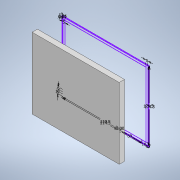
# Autodesk Inventor part: controller_box
Saved by Autodesk Inventor 2022 (Build 260153000, 153)
## iProperties
Created: 2021-07-22
Part Number: controller_box
Material: Generic
Document SubType Name: Modeling
Designer: alibe
Density: 1 g/cm^3
Appearance: Default
Author: alibe
Autodesk Inventor part; units mm, degrees
ref_plane "YZ Plane" through (0, 0, 0) normal (1, 0, 0) x (0, 1, 0)
ref_plane "XZ Plane" through (0, 0, 0) normal (0, 1, 0) x (-1, 0, 0)
ref_plane "XY Plane" through (0, 0, 0) normal (0, 0, 1) x (1, 0, 0)
sketch "Base" plane through (0, 0, 0) normal (0, 0, 1) x (1, 0, 0)
  line L0 (-100, 100) -> (-100, -50)
  line L1 (100, 100) -> (100, -50)
  line L2 (-100, 100) -> (-100, 110)
  line L3 (-100, 110) -> (100, 110)
  line L4 (100, 110) -> (100, 100)
  line L5 (-100, 110) -> (-105, 110)
  line L6 (-105, 110) -> (-105, -50)
  line L7 (-105, -50) -> (-100, -50)
  line L8 (-105, -50) -> (-105, -45)
  line L9 (100, 110) -> (100, 105)
  line L10 (100, 105) -> (-105, 105)
  line L11 (100, 110) -> (105, 110)
  line L12 (105, 110) -> (105, -50)
  line L13 (-105, -50) -> (-105, -60)
  line L14 (-105, -60) -> (105, -60)
  line L15 (105, -60) -> (105, -50)
  line L16 (-105, -60) -> (-105, -55)
  line L17 (-105, -55) -> (105, -55)
  line L18 (100, -50) -> (100, -55)
  line L19 (-100, -50) -> (-100, -55)
  line L20 (-100, -55) -> (-90, -55)
  line L21 (-90, -55) -> (-90, -60)
  line L22 (100, -55) -> (90, -55)
  line L23 (90, -55) -> (90, -60)
  line L24 (-90, -55) -> (-30, -55)
  line L25 (-30, -55) -> (-30, -60)
  line L26 (90, -55) -> (30, -55)
  line L27 (30, -55) -> (30, -60)
  line L28 (-30, -55) -> (-30, 0)
  line L29 (-90, -55) -> (-90, 0)
  line L30 (-90, 0) -> (-30, 0)
  line L31 (30, -55) -> (30, 0)
  line L32 (30, 0) -> (90, 0)
  line L33 (90, 0) -> (90, -55)
  line L34 (-30, -55) -> (-28, -55)
  line L35 (-28, -55) -> (-28, 0)
  line L36 (30, -55) -> (28, -55)
  line L37 (28, -55) -> (28, 0)
  line L38 (-60, -55) -> (-60, 0)
  line L39 (0, 105) -> (0, -55)
  line L40 (-60, 0) -> (-80, 0)
  line L41 (-80, 0) -> (-80, -55)
  line L42 (-60, -55) -> (-40, -55)
  line L43 (-40, -55) -> (-40, 0)
  line L44 (60, -55) -> (60, 0)
  line L45 (80, 0) -> (80, -55)
  line L46 (40, -55) -> (40, 0)
  line L47 (90, -55) -> (95, -55)
  line L48 (80, 0) -> (85, 0)
  line L49 (85, 0) -> (85, -55)
  line L50 (40, -55) -> (35, -55)
  line L51 (35, -55) -> (35, 0)
  line L52 (-85, 0) -> (-85, -55)
  line L53 (-35, -55) -> (-35, 0)
  line L54 (-90, -55) -> (-90, -50)
  line L55 (90, -55) -> (90, -45)
  line L56 (90, -45) -> (28, -45)
  line L57 (-28, -55) -> (-28, -45)
  line L58 (-28, -45) -> (-90, -45)
  line L59 (-90, -45) -> (-90, -35)
  line L60 (-90, -35) -> (-28, -35)
  line L61 (28, -45) -> (28, -35)
  line L62 (28, -35) -> (90, -35)
  point P0 (0, 0)
  point P1 (-100, 105)
  point P2 (-35, -45)
  point P3 (-85, -45)
  point P4 (85, -45)
  point P5 (35, -45)
  point P6 (-85, -35)
  point P7 (-35, -35)
  point P8 (35, -35)
  point P9 (85, -35)
  dimension "d7" = 10
  dimension "d8" = 5
  dimension "d9" = 5
  dimension "d11" = 5
  dimension "d12" = 10
  dimension "d13" = 5
  dimension "d14" = 10
  dimension "d15" = 10
  dimension "d16" = 60
  dimension "d17" = 60
  dimension "d18" = 90
  dimension "d19" = 2
  dimension "d20" = 2
  dimension "d21" = 20
  dimension "d22" = 20
  dimension "d25" = 5
  dimension "d26" = 5
  dimension "d145" = 10
  dimension "d146" = 10
  constraints: 124 end point, 28 point on line, 20 perpendicular, 10 symmetric about line, 8 vertical, 6 midpoint, 1 horizontal, 1 parallel, 12 other
  measures "d7" distance of L0.start L2.end
  measures "d8" distance of L2.end L5.end
  measures "d9" distance of L6.end L8.end
  measures "d11" distance of L3.end L11.end
  measures "d12" distance of L6.end L13.end
  measures "d13" distance of L13.end L16.end
  measures "d14" distance of L19.end L20.end
  measures "d15" distance of L18.end L22.end
  measures "d16" distance of L20.end L24.end
  measures "d17" distance of L22.end L26.end
  measures "d18" angle of L27 L26
  measures "d19" distance of L24.end L34.end
  measures "d20" distance of L26.end L36.end
  measures "d21" distance of L38.end L40.end
  measures "d22" distance of L38.start L42.end
  measures "d25" distance of L45.start L48.end
  measures "d26" distance of L46.start L50.end
  measures "d145" distance of L58.end L59.end
  measures "d146" distance of L56.end L61.end
extrude "base_extrusion" add sketch "Base" against normal blind 3
extrude "wall_extrusion" add sketch "Base" along normal blind 70 contours L0 L7 L6 L10 L2 | L19 L17 L13 L7 | L10 L6 L5 L2 | L2 L3 L4 L10 | L17 L21 L14 L13 | L17 L25 L14 L21 | L11 L12 L15 L17 L18 L1 L4 | L17 L27 L14 L25 | L17 L23 L14 L27 | L15 L14 L23 L17
sketch "pump_holder" plane through (-105, -60, -3) normal (0, -1, 0) x (1, 0, 0)
  line L0 (210, 0) -> (0, 0) projected
  line L1 (0, 73) -> (210, 73)
  line L2 (210, 73) -> (210, 0)
  line L3 (210, 0) -> (0, 0)
  line L4 (0, 0) -> (0, 73)
  line L5 (0, 0) -> (0, 73) projected
  line L6 (0, 0) -> (0, 3)
  line L7 (0, 3) -> (210, 3)
  line L8 (210, 73) -> (210, 0) projected
  line L9 (0, 3) -> (5, 3)
  line L10 (5, 3) -> (5, 0)
  line L11 (5, 3) -> (15, 3)
  line L12 (5, 3) -> (15, 3) construction
  line L13 (15, 3) -> (15, 0)
  line L14 (15, 3) -> (75, 3)
  line L15 (15, 3) -> (75, 3) construction
  line L16 (75, 3) -> (75, 0)
  line L17 (75, 0) -> (77, 0)
  line L18 (15, 0) -> (45, 0)
  line L19 (45, 0) -> (45, 8)
  arc A0 (25, 28) -> (65, 28) centre (45, 28) ccw projected
  line L20 (45, 8) -> (45, 28)
  circle A1 centre (45, 28) radius 20
  line L21 (105, 3) -> (105, 0)
  line L22 (45, 8) -> (45, 10.25)
  line L23 (45, 8) -> (47.25, 8) construction
  line L24 (45, 10.25) -> (74, 10.25)
  line L25 (45, 10.25) -> (73.875, 10.25)
  line L26 (73.875, 10.25) -> (73.875, 55)
  line L27 (73.875, 10.25) -> (118.625, 10.25) construction
  line L28 (73.875, 55) -> (16.125, 55)
  line L29 (73.875, 55) -> (131.625, 55) construction
  line L30 (16.125, 55) -> (16.125, 10.25)
  line L31 (16.125, 10.25) -> (45, 10.25)
  line L32 (45, 28) -> (65, 28)
  line L33 (16.125, 55) -> (16.125, 52)
  line L34 (16.125, 52) -> (19.125, 52)
  line L35 (19.125, 52) -> (20.875, 52)
  line L36 (19.125, 52) -> (20.875, 52) construction
  line L37 (20.875, 52) -> (20.875, 50.25)
  line L38 (20.875, 52) -> (22.625, 52) construction
  line L39 (16.125, 10.25) -> (16.125, 32.625)
  line L40 (16.125, 32.625) -> (21.625, 32.625)
  line L41 (105, 3) -> (105, 73)
  line L42 (205, 73) -> (5, 73) projected
  line L43 (105, 3) -> (175, 3) construction
  line L44 (16.125, 10.25) -> (16.125, 3)
  line L45 (73.875, 10.25) -> (73.875, 3)
  line L46 (20.875, 50.25) -> (20.875, 51.25)
  circle A2 centre (20.875, 51.25) radius 2
  line L47 (21.625, 32.625) -> (22.625, 32.625)
  line L48 (22.625, 32.625) -> (22.625, 33.625)
  circle A3 centre (22.625, 33.625) radius 2
  circle A4 centre (69.125, 51.25) radius 2
  circle A5 centre (67.375, 33.625) radius 2
  line L49 (20.875, 14) -> (20.875, 15)
  circle A6 centre (20.875, 15) radius 2
  circle A7 centre (69.125, 15) radius 2
  circle A8 centre (165, 28) radius 20
  line L50 (165, 10.25) -> (136, 10.25)
  line L51 (165, 10.25) -> (136.125, 10.25)
  line L52 (136.125, 10.25) -> (136.125, 55)
  line L53 (136.125, 55) -> (193.875, 55)
  line L54 (193.875, 55) -> (193.875, 10.25)
  line L55 (193.875, 10.25) -> (165, 10.25)
  line L56 (165, 28) -> (145, 28)
  line L57 (193.875, 55) -> (193.875, 52)
  line L58 (193.875, 52) -> (190.875, 52)
  line L59 (190.875, 52) -> (189.125, 52)
  line L60 (190.875, 52) -> (189.125, 52) construction
  line L61 (189.125, 52) -> (189.125, 50.25)
  line L62 (189.125, 52) -> (187.375, 52) construction
  line L63 (193.875, 10.25) -> (193.875, 32.625)
  line L64 (193.875, 32.625) -> (188.375, 32.625)
  line L65 (189.125, 50.25) -> (189.125, 51.25)
  circle A9 centre (189.125, 51.25) radius 2
  line L66 (188.375, 32.625) -> (187.375, 32.625)
  line L67 (187.375, 32.625) -> (187.375, 33.625)
  circle A10 centre (187.375, 33.625) radius 2
  circle A11 centre (140.875, 51.25) radius 2
  circle A12 centre (142.625, 33.625) radius 2
  line L68 (189.125, 14) -> (189.125, 15)
  circle A13 centre (189.125, 15) radius 2
  circle A14 centre (140.875, 15) radius 2
  point P0 (16.125, 3)
  point P1 (185, 28)
  dimension "d43" = 5
  dimension "d44" = 10
  dimension "d45" = 0
  dimension "d46" = 60
  dimension "d47" = 0
  dimension "d49" = 30
  dimension "d50" = 20
  dimension "d53" = 2.25
  dimension "d54" = 90
  dimension "d56" = 90
  dimension "d58" = 28.875
  dimension "d59" = 44.75
  dimension "d60" = 90
  dimension "d61" = 57.75
  dimension "d62" = 180
  dimension "d63" = 44.75
  dimension "d64" = 90
  dimension "d65" = 3
  dimension "d66" = 3
  dimension "d67" = 90
  dimension "d68" = 1.75
  dimension "d69" = 0
  dimension "d70" = 1.75
  dimension "d71" = 90
  dimension "d72" = 22.375
  dimension "d73" = 5.5
  dimension "d77" = 90
  dimension "d117" = 1
  dimension "d118" = 4
  dimension "d120" = 1
  dimension "d121" = 4
  dimension "d124" = 4
  constraints: 130 end point, 37 symmetric about line, 16 point on line, 14 centre point, 13 horizontal, 12 perpendicular, 10 coincident, 8 equal length, 4 midpoint, 3 vertical, 2 collinear, 2 parallel, 1 concentric, 1 point on circle, 10 other
  measures "d43" distance of L6.end L9.end
  measures "d44" distance of L9.end L11.end
  measures "d45" distance between parallel lines of L11 L12
  measures "d46" distance of L12.end L14.end
  measures "d47" distance between parallel lines of L14 L15
  measures "d49" distance of L13.end L18.end
  measures "d50" distance of L19.end L20.end
  measures "d53" distance of L19.end L22.end
  measures "d54" angle of L23 L22
  measures "d56" angle of L22 L24
  measures "d58" distance of L22.end L25.end
  measures "d59" distance of L25.end L26.end
  measures "d60" angle of L27 L26
  measures "d61" distance of L26.end L28.end
  measures "d62" angle of L28 L29
  measures "d63" distance of L28.end L30.end
  measures "d64" angle of L30 L28
  measures "d65" distance of L28.end L33.end
  measures "d66" distance of L33.end L34.end
  measures "d67" angle of L34 L33
  measures "d68" distance of L34.end L35.end
  measures "d69" distance between parallel lines of L35 L36
  measures "d70" distance of L36.end L37.end
  measures "d71" angle of L37 L38
  measures "d72" distance of L30.end L39.end
  measures "d73" distance of L39.end L40.end
  measures "d77" angle of L43 L41
  measures "d117" distance of L46.start L46.end
  measures "d118" diameter of A2
  measures "d120" distance of L48.start L48.end
  measures "d121" diameter of A3
  measures "d124" diameter of A6
extrude "Extrusion6" cut sketch "pump_holder" against normal blind 5 contours L20 L24 A0 | A0 L31 L20 | L24 L20 L32 A0 | A0 A1 L32 L20 L31
extrude "Extrusion9" add sketch "Base" along normal blind 25 separate body contours L52 L60 L41 L58 | L41 L60 L38 L58 | L52 L30 L41 L60 | L38 L60 L43 L58 | L41 L30 L38 L60 | L58 L43 L60 L53 | L51 L62 L46 L56 | L38 L30 L43 L60 | L60 L43 L30 L53 | L46 L62 L44 L56 | L51 L32 L46 L62 | L44 L62 L45 L56 | L46 L32 L44 L62 | L56 L45 L62 L49 | L44 L32 L45 L62 | L62 L45 L32 L49
sketch "pump_support" plane through (35, 0, 0) normal (0, 1, 0) x (1, 0, 0)
  line L0 (0, 0) -> (50, 0) projected
  line L1 (50, 0) -> (25, 0)
  line L2 (25, 0) -> (25, -5)
  line L3 (25, -5) -> (25, -25)
  line L4 (0, -25) -> (50, -25) projected
  line L5 (45, -25) -> (5, -25)
  arc A0 (45, -25) -> (5, -25) centre (25, -25) ccw
  point P0 (-35, 0)
  dimension "d82" = 5
  constraints: 8 end point, 3 point on circle, 2 midpoint, 2 point on line, 1 centre point, 1 vertical
  measures "d82" distance of L1.end L2.end
extrude "Extrusion10" cut sketch "pump_support" against normal blind 45 bodies 2
sketch "Sketch6" plane through (-85, 0, 0) normal (0, 1, 0) x (1, 0, 0)
  line L0 (0, 0) -> (50, 0)
  line L1 (50, 0) -> (25, 0)
  line L2 (25, 0) -> (25, -5)
  line L3 (25, -5) -> (25, -25)
  line L4 (0, -25) -> (50, -25)
  line L5 (45, -25) -> (5, -25)
  arc A0 (45, -25) -> (5, -25) centre (25, -25) ccw
  point P0 (85, 0)
  point P1 (-35, 0)
  dimension "d86" = 5
  constraints: 12 end point, 3 point on circle, 2 midpoint, 2 point on line, 1 centre point, 1 vertical
  measures "d86" distance of L1.end L2.end
extrude "Extrusion11" cut sketch "Sketch6" against normal blind 45 bodies 2
combine bodies "Combine1" operation type add bodies to combine 1 2
sketch "pH hole" plane through (-105, 110, -3) normal (0, 1, 0) x (1, 0, 0)
  line L0 (210, 0) -> (210, -3)
  line L1 (210, -73) -> (210, 0) projected
  line L2 (210, -3) -> (0, -3)
  line L3 (210, 0) -> (0, 0) projected
  line L4 (0, -3) -> (0, 0)
  line L5 (0, 0) -> (210, 0)
  line L6 (210, -73) -> (0, -73)
  line L7 (0, -73) -> (0, -3)
  line L8 (0, -3) -> (210, -3)
  line L9 (210, -3) -> (210, -73)
  line L10 (5, -3) -> (205, -3) projected
  line L11 (210, -3) -> (205, -3)
  line L12 (205, -3) -> (205, 0)
  line L13 (205, -3) -> (205, -73) projected
  line L14 (205, -3) -> (205, -73)
  line L15 (0, 0) -> (0, -73) projected
  line L16 (0, -3) -> (5, -3)
  line L17 (5, -3) -> (5, 0)
  line L18 (5, -3) -> (5, -73)
  line L19 (205, -3) -> (205, -6.75)
  line L20 (205, -6.75) -> (185, -6.75)
  line L21 (185, -6.75) -> (185, -3)
  line L22 (190, -3) -> (140, -3) projected
  line L23 (185, -6.75) -> (185, -19.25)
  line L24 (185, -19.25) -> (185, -13)
  circle A0 centre (185, -13) radius 6.25
  line L25 (205, -3) -> (205, -38)
  line L26 (205, -38) -> (140, -38)
  line L27 (140, -3) -> (140, -28) projected
  line L28 (140, -38) -> (140, -3)
  circle A1 centre (140, -38) radius 6.25
  circle A2 centre (140, -38) radius 7
  line L29 (5, -3) -> (5, -73) projected
  line L30 (5, -3) -> (5, -38)
  line L31 (5, -38) -> (82.55, -38)
  circle A3 centre (82.55, -38) radius 6.25
  circle A4 centre (82.55, -38) radius 7
  point P0 (105, -3)
  dimension "d127" = 3
  dimension "d128" = 210
  dimension "d129" = 5
  dimension "d130" = 5
  dimension "d131" = 3.75
  dimension "d132" = 20
  dimension "d133" = 12.5
  dimension "d134" = 6.25
  dimension "d137" = 35
  dimension "d138" = 12.5
  dimension "d139" = 14
  dimension "d140" = 14
  constraints: 48 end point, 10 perpendicular, 8 point on line, 5 coincident, 4 centre point, 4 equal length, 3 midpoint, 1 horizontal, 1 vertical alignment, 2 other
  measures "d127" distance of L0.start L0.end
  measures "d128" distance of L2.end L8.end
  measures "d129" distance of L8.end L10.end
  measures "d130" distance of L2.end L10.start
  measures "d131" distance of L10.end L19.end
  measures "d132" distance of L19.end L20.end
  measures "d133" distance of L20.end L23.end
  measures "d134" distance of L23.end L24.end
  measures "d137" distance of L10.end L25.end
  measures "d138" diameter of A1
  measures "d139" diameter of A2
  measures "d140" diameter of A4
extrude "Extrusion18" cut sketch "pH hole" against normal blind 5 contours A1 L28 L26 | L26 L28 A1 | A3 bodies 1
extrude "Extrusion19" cut sketch "pump_holder" against normal blind 5 contours A2 | A3 | A4 | A5 | A6 | A7 | A8 L55 L50 | A8 L50 L55 | A9 | A10 | A11 | A12 | A13 | A14 bodies 1
extrude "Extrusion20" cut sketch "Base" along normal blind 25 contours L52 L60 L41 L58 | L41 L60 L38 L58 | L38 L60 L43 L58 | L58 L43 L60 L53 | L51 L62 L46 L56 | L46 L62 L44 L56 | L44 L62 L45 L56 | L56 L45 L62 L49 bodies 1
sketch "Sketch9" plane through (0, 0, 0) normal (0, 0, 1) x (1, 0, 0)
  line L0 (-100, 100) -> (-100, -50)
  line L1 (100, 100) -> (100, -50)
  line L2 (-100, 100) -> (-100, 110)
  line L3 (-100, 110) -> (100, 110)
  line L4 (100, 110) -> (100, 100)
  line L5 (-100, 110) -> (-105, 110)
  line L6 (-105, 110) -> (-105, -50)
  line L7 (-105, -50) -> (-100, -50)
  line L8 (-105, -50) -> (-105, -45)
  line L9 (100, 110) -> (100, 105)
  line L10 (100, 105) -> (-105, 105)
  line L11 (100, 110) -> (105, 110)
  line L12 (105, 110) -> (105, -50)
  line L13 (-105, -50) -> (-105, -60)
  line L14 (-105, -60) -> (105, -60)
  line L15 (105, -60) -> (105, -50)
  line L16 (-105, -60) -> (-105, -55)
  line L17 (-105, -55) -> (105, -55)
  line L18 (100, -50) -> (100, -55)
  line L19 (-100, -50) -> (-100, -55)
  line L20 (-100, -55) -> (-90, -55)
  line L21 (-90, -55) -> (-90, -60)
  line L22 (100, -55) -> (90, -55)
  line L23 (90, -55) -> (90, -60)
  line L24 (-90, -55) -> (-30, -55)
  line L25 (-30, -55) -> (-30, -60)
  line L26 (90, -55) -> (30, -55)
  line L27 (30, -55) -> (30, -60)
  line L28 (-30, -55) -> (-28, -55)
  line L29 (30, -55) -> (28, -55)
  line L30 (-60, -55) -> (-40, -55)
  line L31 (90, -55) -> (95, -55)
  line L32 (40, -55) -> (35, -55)
  line L33 (-105, 110) -> (-105, 110.25)
  line L34 (-105, 110.25) -> (-105.25, 110.25)
  line L35 (-105.25, 110.25) -> (105.25, 110.25)
  line L36 (105.25, 110.25) -> (105.25, -60.25)
  line L37 (105.25, -60.25) -> (-105.25, -60.25)
  line L38 (-105.25, -60.25) -> (-105.25, 110.25)
  line L39 (-105.25, 110.25) -> (-105.25, 112.25)
  line L40 (-105.25, 112.25) -> (-107.25, 112.25)
  line L41 (-107.25, 112.25) -> (107.25, 112.25)
  line L42 (107.25, 112.25) -> (107.25, -62.25)
  line L43 (107.25, -62.25) -> (-107.25, -62.25)
  line L44 (-107.25, -62.25) -> (-107.25, 112.25)
  point P0 (-35, 0)
  point P1 (-85, 0)
  point P2 (-100, 105)
  point P3 (-85, -55)
  point P4 (-35, -55)
  point P5 (40, 0)
  point P6 (-35, -45)
  point P7 (-85, -45)
  point P8 (85, -45)
  point P9 (35, -45)
  point P10 (-85, -35)
  point P11 (-35, -35)
  point P12 (35, -35)
  point P13 (85, -35)
  dimension "d149" = 10
  dimension "d150" = 5
  dimension "d151" = 5
  dimension "d152" = 5
  dimension "d153" = 10
  dimension "d154" = 5
  dimension "d156" = 10
  dimension "d158" = 60
  dimension "d159" = 90
  dimension "d161" = 2
  dimension "d165" = 5
  dimension "d168" = 0.25
  dimension "d169" = 0.25
  dimension "d170" = 210.5
  dimension "d171" = 170.5
  dimension "d172" = 2
  dimension "d173" = 2
  dimension "d174" = 214.5
  dimension "d175" = 174.5
  constraints: 88 end point, 15 perpendicular, 10 point on line, 5 midpoint, 5 vertical, 4 parallel, 3 horizontal, 11 other
  measures "d149" distance of L0.start L2.end
  measures "d150" distance of L2.end L5.end
  measures "d151" distance of L6.end L8.end
  measures "d152" distance of L3.end L11.end
  measures "d153" distance of L6.end L13.end
  measures "d154" distance of L13.end L16.end
  measures "d156" distance of L18.end L22.end
  measures "d158" distance of L22.end L26.end
  measures "d159" angle of L27 L26
  measures "d161" distance of L26.end L29.end
  measures "d165" distance of L32.start L32.end
  measures "d168" distance of L5.end L33.end
  measures "d169" distance of L33.end L34.end
  measures "d170" distance of L36.end L37.end
  measures "d171" distance of L35.end L36.end
  measures "d172" distance of L34.end L39.end
  measures "d173" distance of L39.end L40.end
  measures "d174" distance of L42.end L43.end
  measures "d175" distance of L41.end L42.end
extrude "Extrusion21" add sketch "Sketch9" along normal blind 3 from surface at 70 separate body contours L2 L10 L4 L1 L18 L17 L19 L0 | L0 L7 L6 L10 L2 | L19 L17 L13 L7 | L10 L6 L5 L2 | L2 L3 L4 L10 | L17 L21 L14 L13 | L4 L11 L12 L15 L17 L18 L1 | L17 L25 L14 L21 | L25 L17 L27 L14 | L17 L15 L14 L23 | L27 L17 L23 L14 | L35 L36 L37 L38 L34 | L41 L42 L43 L44 L40
extrude "Extrusion22" add sketch "Sketch9" against normal blind 10 from surface at 70 separate body contours L41 L42 L43 L44 L40
combine bodies "Combine2" operation type add bodies to combine 3 4
